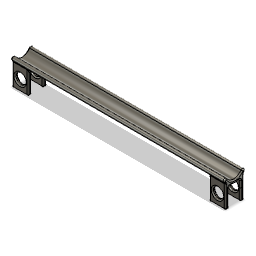
Ball Slider (Autodesk Fusion 360 design; units mm, degrees)
Autodesk Fusion 360 part; units mm, degrees
sketch "Sketch1" plane through (0, 0, 0) normal (1, 0, 0) x (0, 0, -1)
  arc A0 (-12.5, 0) -> (12.5, 0) centre (0, 7.660714) ccw
  arc A1 (-17.615713, -3.135201) -> (17.615713, -3.135201) centre (0, 7.660714) ccw
  arc A2 (-12.5, 0) -> (-17.615713, -3.135201) centre (-15.057856, -1.5676) ccw
  arc A3 (17.615713, -3.135201) -> (12.5, 0) centre (15.057856, -1.5676) ccw
  point P0 (0, -7)
  dimension "d7" = 25
  dimension "d8" = 12.5
  dimension "d9" = 7
  constraint horizontal A0.start A0.end
  constraint coincident P0 A0
  constraint coincident A0.end A3.end
  constraint coincident A0.start A2.start
  constraint tangent A1 A2
  constraint concentric A0 A1
  constraint tangent A1 A3
  measures "d7" distance of A0.start A0.end
  measures "d8" distance of origin A0.start
  measures "d9" distance of origin P0
extrude "Extrude1" add sketch "Sketch1" along normal blind 370
sketch "Sketch2" plane through (370, 0, 0) normal (1, 0, 0) x (0, 0, -1)
  arc A0 (-12.5, 0) -> (-17.615713, -3.135201) centre (-15.057856, -1.5676) ccw
  arc A1 (-17.615713, -3.135201) -> (17.615713, -3.135201) centre (0, 7.660714) ccw
  arc A2 (17.615713, -3.135201) -> (12.5, 0) centre (15.057856, -1.5676) ccw
  arc A3 (-12.5, 0) -> (12.5, 0) centre (0, 7.660714) ccw
  line L0 (-16, -5) -> (-10, -5)
  line L1 (-10, -5) -> (-10, -25)
  line L2 (-16, -25) -> (-16, -5)
  line L3 (-10, -10.418697) -> (-10, -45.418697)
  line L4 (-16, -25) -> (-16, -45.418697)
  line L5 (-16, -45.418697) -> (-10, -45.418697)
  line L6 (0, 15) -> (0, -55.000001) construction
  line L7 (10, -10.418697) -> (10, -45.418697)
  line L8 (16, -45.418697) -> (10, -45.418697)
  line L9 (16, -25) -> (16, -45.418697)
  line L10 (16, -25) -> (16, -5)
  line L11 (16, -5) -> (10, -5)
  line L12 (10, -5) -> (9.999999, -25)
  point P0 (-10, -10.418697)
  dimension "d14" = 6
  dimension "d15" = 20
  dimension "d16" = 35
  dimension "d21" = 10
  dimension "d22" = 10
  constraint horizontal L0
  constraint vertical L1
  constraint vertical L2
  constraint parallel L1 L3
  constraint perpendicular L3 L5
  constraint vertical L6
  constraint symmetric L0.start L6 L10.end
  constraint symmetric L0.end L6 L11.end
  constraint symmetric L2.start L6 L9.start
  measures "d14" distance of L0.start L0.end
  measures "d15" distance of L0.start L2.start
  measures "d21" distance of origin L12
  measures "d22" distance of L3 L6
extrude "Extrude2" add sketch "Sketch2" against normal blind 28 contours A1 L1 L2 L3 L4 L5 | A1 L7 L8 L9 L10 L12 picked at (-14, -31.806232) picked at (12, -31.806232)
fillet "Fillet1" radius 2 30 edges at (370, -4.300325, -16.846324) (370, 0.990256, -16.625457) (370, -7, 0) (370, 0.990256, 16.625457) (370, -4.300325, 16.846325) (370, -13, 0) (370, -27.918697, 10) (370, -25.41476, 16) (370, -17.709349, -9.999999) (370, -35.209349, -9.999999) (370, -25.414761, -16) (370, -45.418697, -13) (370, -45.418697, 13) (356, -10.418697, 10) (356, -10.418697, -10) (342, -25.41476, 16) (342, -27.918697, 10) (356, -45.418697, 16) (356, -45.418697, 10) (356, -45.418697, -10) (356, -45.418697, -16) (342, -25.414761, -16) (342, -35.209349, -9.999999) (342, -17.709349, -9.999999) (342, -45.418697, -13) (342, -45.418697, 13) (356, -5.410824, 16) (356, -5.410824, -16) (342, -8.201046, -13.238946) (342, -8.201045, 13.238946)
sketch "Sketch3" plane through (0, 0, 16) normal (0, 0, 1) x (1, 0, 0)
  line L0 (368, -38.418697) -> (368, -6.105475)
  line L1 (368, -6.105475) -> (344, -6.105475)
  line L2 (344, -6.105475) -> (344, -38.418697)
  line L3 (344, -38.418697) -> (368, -38.418697)
  circle A0 centre (356, -26.418697) radius 9
  dimension "d23" = 24
  dimension "d24" = 32.313222
  dimension "d25" = 18
  dimension "d30" = 12
  measures "d25" diameter of A0
extrude "Extrude3" cut sketch "Sketch3" against normal up to surface (32 mm away) contours A0 picked at (353.70107, -23.046786)
fillet "Fillet2" radius 2 5 edges at (347.609054, -23.164158, 16) (347.609054, -29.673236, 10) (356, -35.418697, -10) (356, -17.418697, -9.999999) (347.609054, -29.673236, -16)
ref_plane "WorkPlane1" through (356, -25.41476, 36) normal (0, 0, 1) x (0, 1, 0)
sketch "Sketch4" plane through (0, 0, 36) normal (0, 0, 1) x (1, 0, 0)
  line L0 (185, 100) -> (185, -100) construction
  line L1 (0, -13) -> (0, -3.135201)
  line L2 (185, 19.161306) -> (0, 19.161306)
  line L3 (0, 19.161306) -> (0, -50)
  line L4 (0, -50) -> (185, -50)
  line L5 (185, -50) -> (185, 19.161306)
  point P0 (370, -2.090134)
  dimension "d32" = 370
  dimension "d33" = 185
  constraint vertical L0
  constraint horizontal L2
  constraint vertical L3
  constraint horizontal L4
  constraint vertical L5
  measures "d33" distance of L0 L1.start
extrude "Extrude4" cut sketch "Sketch4" against normal blind 200
mirror "Mirror1" about plane through (185, -50, 36) normal (-1, 0, 0) of bodies 1 merged
equation "d8 = ( 25 / 2 ) * 1 mm"
equation "d33 = ( 370 / 2 ) * 1 mm"
